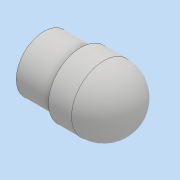
# Autodesk Inventor part: P7
Saved by Autodesk Inventor 2017 (Build 210142000, 142)
## iProperties
Part Number: P7
Material: 一般
Document SubType Name: Modeling
Designer: d8910
Density: 1 g/cm^3
Appearance: 預設
Author: d8910
Autodesk Inventor part; units mm, degrees
ref_plane "YZ Plane" through (0, 0, 0) normal (1, 0, 0) x (0, 1, 0)
ref_plane "XZ Plane" through (0, 0, 0) normal (0, 1, 0) x (-1, 0, 0)
ref_plane "XY Plane" through (0, 0, 0) normal (0, 0, 1) x (1, 0, 0)
sketch "草圖1" plane through (0, 0, 0) normal (0, 0, 1) x (1, 0, 0)
  line L0 (-32.5, 0) -> (-12.5, 0)
  line L1 (-12.5, 0) -> (-12.5, 15)
  line L2 (-12.5, 15) -> (-32.5, 15)
  line L3 (-32.5, 15) -> (-32.5, 0)
  line L4 (-12.5, 0) -> (17.5, 0)
  line L5 (0, 0) -> (0, 17.5)
  line L6 (0, 17.5) -> (-12.5, 17.5)
  line L7 (-12.5, 17.5) -> (-12.5, 0)
  arc A0 (17.5, 0) -> (0, 17.5) centre (0, 0) ccw
  dimension "d0" = 50
  dimension "d1" = 15
  dimension "d2" = 20
  dimension "d3" = 17.5
  constraints: 16 end point, 4 parallel, 2 coincident, 2 horizontal, 2 perpendicular, 2 point on circle, 1 centre point, 1 point on line, 1 vertical alignment
  measures "d0" distance from line of L3 L4.end
  measures "d1" distance between parallel lines of L0 L2
  measures "d2" distance of L1.end L2.end
  measures "d3" radius of A0
revolve "迴轉1" add sketch "草圖1" angle 360 about axis through (-12.5, 0, 0) along (1, 0, 0)
